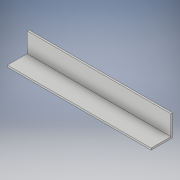
# Autodesk Inventor part: CLB_061_OutsideLBracket
Saved by Autodesk Inventor 2018.3 (Build 223284000, 284)
## iProperties
Created: 2020-02-17
Part Number: CLB_061_OutsideLBracket
Material: Generic
Document SubType Name: Modeling
Designer: 22perngrac
Density: 1 g/cm^3
Appearance: Default
Author: 22perngrac
Autodesk Inventor part; units mm, degrees
ref_plane "YZ Plane" through (0, 0, 0) normal (1, 0, 0) x (0, 1, 0)
ref_plane "XZ Plane" through (0, 0, 0) normal (0, 1, 0) x (-1, 0, 0)
ref_plane "XY Plane" through (0, 0, 0) normal (0, 0, 1) x (1, 0, 0)
sketch "Sketch1" plane through (0, 0, 0) normal (0, 0, 1) x (1, 0, 0)
  line L0 (0, 0) -> (254, 0)
  line L1 (254, 0) -> (254, 38.1)
  line L2 (254, 38.1) -> (0, 38.1)
  line L3 (0, 38.1) -> (0, 0)
  dimension "d0" = 254
  dimension "d1" = 38.1
  constraints: 8 end point, 2 parallel, 1 horizontal, 1 perpendicular
  measures "d0" distance of L1.end L2.end
  measures "d1" distance of L0.end L1.end
extrude "Extrusion1" add sketch "Sketch1" along normal blind 3.175
sketch "Sketch2" plane through (0, 0, 3.175) normal (0, 0, 1) x (1, 0, 0)
  line L0 (0, 0) -> (254, 0) projected
  line L1 (0, 0) -> (254, 0)
  line L2 (254, 0) -> (254, 3.175)
  line L3 (254, 3.175) -> (0, 3.175)
  line L4 (0, 3.175) -> (0, 0)
  dimension "d4" = 3.175
  dimension "d5" = 254
  constraints: 8 end point, 2 parallel, 1 horizontal, 1 perpendicular
  measures "d4" distance of L1.end L2.end
  measures "d5" distance of L2.end L3.end
extrude "Extrusion2" add sketch "Sketch2" along normal blind 34.925
body "Solid1"
